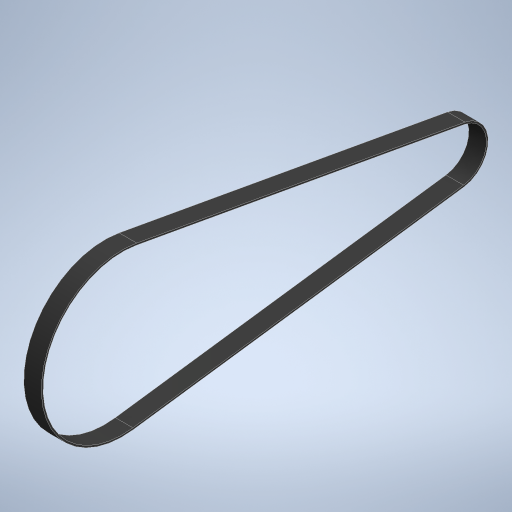
# Autodesk Inventor part: type5
Saved by Autodesk Inventor 2023 (Build 270158000, 158)
## iProperties
Created: 2022-04-24
Part Number: type5
Material: ゴム
Document SubType Name: Modeling
Designer: yuta
Density: 0.93 g/cm^3
Appearance: ゴム - 黒
Author: yuta
Autodesk Inventor part; units mm, degrees
ref_plane "YZ Plane" through (0, 0, 0) normal (1, 0, 0) x (0, 1, 0)
ref_plane "XZ Plane" through (0, 0, 0) normal (0, 1, 0) x (-1, 0, 0)
ref_plane "XY Plane" through (0, 0, 0) normal (0, 0, 1) x (1, 0, 0)
sketch "スケッチ1" plane through (0, 0, 0) normal (1, 0, 0) x (0, 1, 0)
  arc A0 (45.2642, -8.1944) -> (-45.5834, -6.1769) centre (0, 0) ccw
  arc A1 (-20.1179, -194.1032) -> (11.4813, -194.8049) centre (-4.2628, -191.9547) ccw
  line L0 (45.2642, -8.1944) -> (11.4813, -194.8049)
  line L1 (-45.5834, -6.1769) -> (-20.1179, -194.1032)
  arc A2 (44.2802, -8.0163) -> (-44.5924, -6.0426) centre (0, 0) ccw
  arc A3 (-19.1269, -193.9689) -> (10.4973, -194.6268) centre (-4.2628, -191.9547) ccw
  line L2 (44.2802, -8.0163) -> (10.4973, -194.6268)
  line L3 (-44.5924, -6.0426) -> (-19.1269, -193.9689)
  dimension "d0" = 92
  dimension "d1" = 32
  dimension "d2" = 192.002
  dimension "d3" = 90
  constraints: 8 end point, 8 point on circle, 8 tangent, 4 centre point, 3 coincident
  measures "d0" diameter of A0
  measures "d1" diameter of A1
  measures "d2" distance of A1.centre point (0, 0)
  measures "d3" diameter of A2
extrude "押し出し1" add sketch "スケッチ1" along normal blind 10
